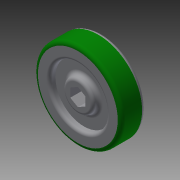
# Autodesk Inventor part: 2338_2015_C_P_M_004_Wheel
Saved by Autodesk Inventor 2015 (Build 190159000, 159)
## iProperties
Created: 2015-01-15
Part Number: 2338_2015_C_P_M_004_Wheel
Material: Generic
Document SubType Name: Modeling
Designer: rickab1
Density: 0.834327 g/cm^3
Appearance: Default
Mass: 143.165 g
Surface Area: 339.571 cm^2
Volume: 171.594 cm^3
Author: rickab1
Autodesk Inventor part; units mm, degrees
ref_plane "YZ Plane" through (0, 0, 0) normal (1, 0, 0) x (0, 1, 0)
ref_plane "XZ Plane" through (0, 0, 0) normal (0, 1, 0) x (-1, 0, 0)
sketch "Sketch1" plane through (0, 0, 0) normal (0, 0, 1) x (1, 0, 0)
  circle A0 centre (0, 0) radius 36.5125
  circle A1 centre (0, 0) radius 23.8125
  dimension "d0" = 73.025
  dimension "d1" = 47.625
  constraints: 2 centre point, 2 coincident
  measures "d0" diameter of A0
  measures "d1" diameter of A1
extrude "Extrusion1" add sketch "Sketch1" along normal blind 20.32 contours A0 | A1
extrude "Extrusion2" cut sketch "Sketch1" along normal blind 5.08 contours A1
fillet "Fillet1" radius 3.175 1 edges at (-36.5125, 0, 20.32)
fillet "Fillet2" radius 2.54 1 edges at (-23.8125, 0, 0)
sketch "Sketch2" plane through (0, 0, 5.08) normal (0, 0, -1) x (-1, 0, 0)
  circle A0 centre (0, 0) radius 23.8125 projected
  circle A1 centre (0, 0) radius 12.7
  dimension "d8" = 25.4
  constraints: 1 centre point, 1 coincident
  measures "d8" diameter of A1
extrude "Extrusion3" add sketch "Sketch2" along normal blind 5.08 contours A1
fillet "Fillet3" radius 3.175 1 edges at (12.7, 0, 5.08)
fillet "Fillet4" radius 2.54 1 edges at (12.7, 0, 0)
ref_plane "Work Plane2" through (0, 0, 10.16) normal (0, 0, -1) x (-1, 0, 0)
mirror "Mirror1" about plane through (0, 0, 10.16) normal (0, 0, -1) of "Extrusion2"
mirror "Mirror2" about plane through (0, 0, 10.16) normal (0, 0, -1) of "Fillet1", "Fillet2"
mirror "Mirror3" about plane through (0, 0, 10.16) normal (0, 0, -1) of "Extrusion3"
mirror "Mirror4" about plane through (0, 0, 10.16) normal (0, 0, -1) of "Fillet3", "Fillet4"
sketch "Sketch3" plane through (0, 0, 0) normal (0, 0, -1) x (-1, 0, 0)
  line L0 (6.35, 3.6662) -> (6.35, -3.6662)
  line L1 (6.35, -3.6662) -> (0, -7.3323)
  line L2 (0, -7.3323) -> (-6.35, -3.6662)
  line L3 (-6.35, -3.6662) -> (-6.35, 3.6662)
  line L4 (-6.35, 3.6662) -> (0, 7.3323)
  line L5 (0, 7.3323) -> (6.35, 3.6662)
  point P0 (10.1954, -0.0083)
  point P1 (0, 0)
  point P2 (0, 0)
  dimension "d13" = 12.7
  constraints: 12 end point, 1 coincident, 1 vertical alignment, 13 other
  measures "d13" distance between parallel lines of L2 L5
extrude "Extrusion4" cut sketch "Sketch3" against normal blind 254
body "Solid1"
